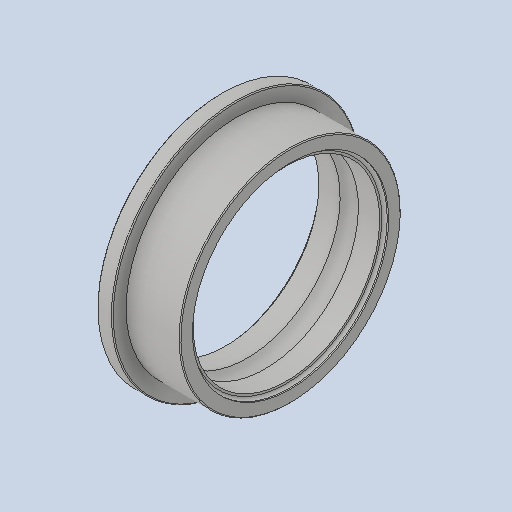
# Autodesk Inventor part: SKF_W 628/8 R-2RS1_PART2
Saved by Autodesk Inventor 2024 (Build 280153000, 153)
## iProperties
Category: PARTsolutions
Company: SKF
Created: 2022-08-03
Part Number: SKF_W 628/8 R-2RS1_PART2
Material: Generic
Catalog Web Link: www.cadenas.de
Description: -Deep groove ball bearings
Vendor: SKF
Document SubType Name: Modeling
Designer: psAdmin
Manufacturer: SKF
Mass: 4 g
Surface Area: 6.88601 cm^2
Volume: 0.330075 cm^3
Density: 1 g/cm^3
Appearance: PSOLRGB-175-175-175
PSOL_IDENT_0: {$CADENAS_DATA/23d-libs/skf/bearings_units_and_housings/ball_bearings/deep_groove_ball_bearings/bb1_
PSOL_IDENT_1: 001_101.prj},215 {VTYP=3D},{NB=SKF_W 628/8 R-2RS1_PART2},{LINA=SKF_W 628/8 R-2RS1_PART2},{NN=BB1_001
PSOL_IDENT_2: _101_PART2},{NOPRJ=TRUE},{DATE=29.07.2022 12:16:16},{GEOMDATE=04.07.2022 10:54:51},{VERSION=},{LINEI
PSOL_IDENT_3: D=22660},{WBVAR=},{WBNUMERIC=}  {NB=SKF_W 628/8 R-2RS1_PART2},{LINA=SKF_W 628/8 R-2RS1_PART2},{KT=DU
PSOL_IDENT_4: MMY},{DESIGNATION=W 628/8 R-2RS1},{R12=0.20},{DD=8.000},{D=16.000},{B=5.000},{C=},{CX=},{CXX=1.1},{C
PSOL_IDENT_5: A=1.100},{XXVARIANT=Flanged outer ring},{XXDESIGN=Single row stainless steel},{XXSEALING=Contact sea
PSOL_IDENT_6: l on both sides},{DESIGN=dgbbwr2zs},{DESIGNIR=dgbbwr2zs},{VARIANT=Flanged outer ring},{DD1=10.50},{D
PSOL_IDENT_7: D2=9.65},{DD2X=},{DD2A=9.65},{D1=13.50},{D1X=0.00},{D2=14.2},{D2A=14.20},{D3=18},{D3X=},{D3A=18.000}
PSOL_IDENT_8: ,{D4=},{HH=0.000},{BB=0.000},{BBX=},{BBA=0.000},{FF=},{R0MAX=0.000},{R0=0.000},{PITCH=12.00},{DW=2.0
PSOL_IDENT_9: 00},{DDAMIN=9.500},{DDAMAX=9.600},{DDBMIN=0.000},{DDBMAX=0.000},{DBMIN=0.000},{DAMAX=0.000},{BBAMIN=
PSOL_IDENT_10: 0.000},{CAMAX=0.000},{RAMAX=0.200},{LOAD1=0.715},{LOAD2=0.300},{LOAD3=0.012},{SPEED1=0},{SPEED2=2600
PSOL_IDENT_11: 0},{KR=0.020},{F0=7.500},{Z=10},{II=1},{MASS=0.004},{BEARING=W 628/8 R-2RS1},{RING=},{HELP=1.250},{H
PSOL_IDENT_12: ELP2=0.900},{DD1ALG=5.250},{YALG=5.250},{PITCH1=12.000},{DW1=2.000},{YALG1=6.750},{HALG1=1.250},{SH=
PSOL_IDENT_13: 4.825},{CU=0.600},{HALG=1.25},{B1=-2.55},{SHIELDHELP=2},{D4A=0.000},{FFA=0.000},{RS1=},{HELP3=0}
NB: SKF_W 628/8 R-2RS1_PART2
NT: Deep groove ball bearings
NBSYN: SKF_$DESIGNATION._PART2
LINA: SKF_W 628/8 R-2RS1_PART2
CATALOG: SKF
DESIGNATION: W 628/8 R-2RS1
R12: 0.2
DD: 8
D: 16
B: 5
XXVARIANT: Flanged outer ring
XXDESIGN: Single row stainless steel
XXSEALING: Contact seal on both sides
DD2: 9.65
D2: 14.2
LOAD1: 0.715
LOAD2: 0.3
LOAD3: 0.012
SPEED1: 0
SPEED2: 26000
BEARING: W 628/8 R-2RS1
SUPPLIER: SKF
ARTICLENO: SKF_W 628/8 R-2RS1_PART2
BOMINFO: SKF_W 628/8 R-2RS1_PART2
CREATOR: CADENAS GmbH
Title: SKF_W 628/8 R-2RS1_PART2
Author: Cadenas PARTsolutions
Comments: Deep groove ball bearings
Autodesk Inventor part; units mm, degrees
ref_plane "YZ Plane" through (0, 0, 0) normal (1, 0, 0) x (0, 1, 0)
ref_plane "XZ Plane" through (0, 0, 0) normal (0, 1, 0) x (-1, 0, 0)
ref_plane "XY Plane" through (0, 0, 0) normal (0, 0, 1) x (1, 0, 0)
sketch "Sketch_21" plane through (0, 0, 0) normal (0, 0, 1) x (1, 0, 0)
  line L0 (50, 0) -> (-50, 0)
  line L1 (0, 8.9333) -> (0, 7.1)
  line L2 (0, 7.1) -> (0.1, 7.1)
  arc A0 (0.3, 6.9) -> (0.1, 7.1) centre (0.1, 6.9) ccw
  line L3 (0.3, 6.9) -> (0.3, 6.75)
  line L4 (0.3, 6.75) -> (1.8386, 6.75)
  arc A1 (3.1614, 6.75) -> (1.8386, 6.75) centre (2.5, 6) ccw
  line L5 (3.1614, 6.75) -> (4.7, 6.75)
  line L6 (4.7, 6.75) -> (4.7, 6.9)
  arc A2 (4.9, 7.1) -> (4.7, 6.9) centre (4.9, 6.9) ccw
  line L7 (4.9, 7.1) -> (5, 7.1)
  line L8 (5, 7.1) -> (5, 7.9333)
  arc A3 (5, 7.9333) -> (4.9333, 8) centre (4.9333, 7.9333) ccw
  line L9 (4.9333, 8) -> (1.1, 8)
  line L10 (1.1, 8) -> (1.1, 8.9333)
  arc A4 (1.1, 8.9333) -> (1.0333, 9) centre (1.0333, 8.9333) ccw
  line L11 (1.0333, 9) -> (0.0667, 9)
  arc A5 (0.0667, 9) -> (0, 8.9333) centre (0.0667, 8.9333) ccw
  constraints: 24 end point, 12 point on circle, 6 centre point
revolve "Revolution1" add sketch "Sketch_21" angle 360 about axis through (50, 0, 0) along (1, 0, 0)
body "Solid1"
